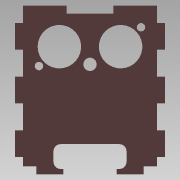
# Autodesk Inventor part: srfdepan
Saved by Autodesk Inventor 2015 SP1 (Build 190203100, 203)
## iProperties
Created: 2015-02-13
Part Number: srfdepan
Material: Generic
Document SubType Name: Modeling
Designer: Rafi Kurnia Putra
Density: 1 g/cm^3
Appearance: Default(1)
Author: Rafi Kurnia Putra
Autodesk Inventor part; units mm, degrees
ref_plane "YZ Plane" through (0, 0, 0) normal (1, 0, 0) x (0, 1, 0)
ref_plane "XZ Plane" through (0, 0, 0) normal (0, 1, 0) x (-1, 0, 0)
ref_plane "XY Plane" through (0, 0, 0) normal (0, 0, 1) x (1, 0, 0)
sketch "Sketch1" plane through (0, 0, 0) normal (0, 0, 1) x (1, 0, 0)
  line L0 (-8.75, -31.5) -> (-25.0209, -31.5)
  line L1 (-8.75, -31.5) -> (-8.75, -28.5)
  line L2 (-8.75, -28.5) -> (8.7497, -28.5)
  line L3 (8.7497, -28.5) -> (8.7497, -31.5)
  line L4 (25.0209, -31.5) -> (8.7497, -31.5)
  circle A0 centre (11.43, -16.1838) radius 8.115
  circle A1 centre (19.05, -8.9448) radius 1.5875
  circle A2 centre (0, -9.5798) radius 2.5
  circle A3 centre (-11.43, -16.1838) radius 8.115
  circle A4 centre (-19.05, -23.4228) radius 1.5875
  line L5 (10.9798, 20.204) -> (-10.9802, 20.204)
  line L6 (13.6378, 26.842) -> (13.6378, 22.862)
  line L7 (-13.6382, 22.862) -> (-13.6382, 26.842)
  arc A5 (-13.6382, 22.862) -> (-10.9802, 20.204) centre (-10.9802, 22.862) ccw
  arc A6 (10.9798, 20.204) -> (13.6378, 22.862) centre (10.9798, 22.862) ccw
  arc A7 (13.6378, 26.842) -> (10.9798, 29.5) centre (10.9798, 26.842) ccw
  arc A8 (-10.9802, 29.5) -> (-13.6382, 26.842) centre (-10.9802, 26.842) ccw
  line L8 (25.0209, -31.5) -> (-25.0209, 31.5) construction
  line L9 (-25.0209, -31.5) -> (25.0209, 31.5) construction
  line L10 (-5, 31.5) -> (5, 31.5)
  line L11 (5, 28.5) -> (-5, 31.5) construction
  line L12 (-5, 28.5) -> (5, 31.5) construction
  line L13 (10, 31.5) -> (20, 31.5)
  line L14 (-20, 31.5) -> (-10, 31.5)
  line L15 (-5, 31.5) -> (5, 31.5)
  line L16 (20, 28.5) -> (25.0209, 28.5)
  line L17 (20, 28.5) -> (20, 31.5)
  line L18 (10, 31.5) -> (10, 28.5)
  line L19 (10, 28.5) -> (5, 28.5)
  line L20 (-5, 28.5) -> (-10, 28.5)
  line L21 (-10, 28.5) -> (-10, 31.5)
  line L22 (-20, 31.5) -> (-20, 28.5)
  line L23 (-20, 28.5) -> (-25.0209, 28.5)
  line L24 (10, 29.5) -> (10.9798, 29.5)
  line L25 (-10.9802, 29.5) -> (-10, 29.5)
  line L26 (28.0209, -5) -> (28.0209, 5)
  line L27 (28.0209, -5) -> (38.0209, -5) construction
  line L28 (0, 0) -> (0, -5) construction
  line L29 (28.0209, -25) -> (28.0209, -15)
  line L30 (28.0209, 15) -> (28.0209, 25)
  line L31 (28.0209, -5) -> (28.0209, 5)
  line L32 (28.0209, -25) -> (25.0209, -25)
  line L33 (28.0209, -15) -> (25.0209, -15)
  line L34 (28.0209, -5) -> (25.0209, -5)
  line L35 (28.0209, 5) -> (25.0209, 5)
  line L36 (28.0209, 15) -> (25.0209, 15)
  line L37 (28.0209, 25) -> (25.0209, 25)
  line L38 (25.0209, -31.5) -> (25.0209, -25)
  line L39 (25.0209, -15) -> (25.0209, -5)
  line L40 (25.0209, 5) -> (25.0209, 15)
  line L41 (25.0209, 25) -> (25.0209, 28.5)
  line L42 (-28.0209, -25) -> (-28.0209, -15)
  line L43 (-28.0209, 15) -> (-28.0209, 25)
  line L44 (-28.0209, -25) -> (-25.0209, -25)
  line L45 (-28.0209, -15) -> (-25.0209, -15)
  line L46 (-28.0209, -5) -> (-25.0209, -5)
  line L47 (-28.0209, 5) -> (-25.0209, 5)
  line L48 (-28.0209, 15) -> (-25.0209, 15)
  line L49 (-28.0209, 25) -> (-25.0209, 25)
  line L50 (-25.0209, -15) -> (-25.0209, -5)
  line L51 (-25.0209, 5) -> (-25.0209, 15)
  line L52 (-25.0209, -31.5) -> (-25.0209, -25)
  line L53 (-25.0209, -15) -> (-25.0209, -5)
  line L54 (-25.0209, 5) -> (-25.0209, 15)
  line L55 (-25.0209, 25) -> (-25.0209, 28.5)
  line L56 (-28.0209, -5) -> (-28.0209, 5)
  line L57 (5, 28.5) -> (-5, 28.5)
  point P0 (0, 0)
  point P1 (0, 30)
  point P2 (35.0209, 0)
  point P3 (-35.0209, 0)
  dimension "d0" = 10
  dimension "d1" = 3
  dimension "d4" = 15
  dimension "d7" = 15
  dimension "d14" = 10
  dimension "d15" = 90
  dimension "d18" = 20
  dimension "d21" = 20
  dimension "d26" = 3
  constraints: 116 end point, 27 perpendicular, 13 symmetric about line, 9 centre point, 8 point on circle, 8 vertical, 6 point on line, 4 horizontal, 3 midpoint, 2 parallel, 1 collinear, 18 other
  measures "d0" distance of L11.start L12.start
  measures "d1" distance of L12.start L10.start
  measures "d4" distance of L10.start L13.start
  measures "d7" distance of L10.start L14.start
  measures "d14" distance of L26.start L26.end
  measures "d15" angle of L27 L26
  measures "d18" distance of L26.start L29.start
  measures "d21" distance of L26.start L30.start
  measures "d26" distance of L29.start L32.end
extrude "Extrusion1" add sketch "Sketch1" along normal mid plane 3 contours L0 L52 L44 L42 L45 L50 L46 L56 L47 L51 L48 L43 L49 L55 L23 L22 L14 L21 L25 A8 L7 A5 L5 A6 L6 A7 L24 L18 L13 L17 L16 L41 L37 L30 L36 L40 L35 L26 L34 L39 L33 L29 L32 L38 L4 L3 L2 L1
body "Solid1"
